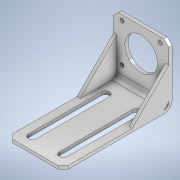
# Autodesk Inventor part: MotorBracket
Saved by Autodesk Inventor 2022 (Build 260153000, 153)
## iProperties
Created: 2022-09-25
Part Number: MotorBracket
Material: Stainless Steel
Document SubType Name: Modeling
Designer: adam
Density: 8 g/cm^3
Appearance: Aluminum - Dark
Mass: 392.424 g
Surface Area: 290.171 cm^2
Volume: 49.053 cm^3
Author: adam
Autodesk Inventor part; units mm, degrees
ref_plane "YZ Plane" through (0, 0, 0) normal (1, 0, 0) x (0, 1, 0)
ref_plane "XZ Plane" through (0, 0, 0) normal (0, 1, 0) x (-1, 0, 0)
ref_plane "XY Plane" through (0, 0, 0) normal (0, 0, 1) x (1, 0, 0)
sketch "Sketch1" plane through (0, 0, 0) normal (1, 0, 0) x (0, 1, 0)
  line L0 (0, 0) -> (4, 0)
  line L1 (4, 6) -> (4, 130)
  line L2 (4, 130) -> (0, 130)
  line L3 (0, 130) -> (0, 0)
  line L4 (10, 0) -> (74, 0)
  line L5 (74, 0) -> (74, -4)
  line L6 (74, -4) -> (10, -4)
  line L7 (0, 6) -> (0, 0)
  line L8 (4, 45) -> (49, 0)
  arc A0 (4, 6) -> (10, 0) centre (10, 6) ccw
  arc A1 (0, 6) -> (10, -4) centre (10, 6) ccw
  line L9 (4, 6) -> (10, 0)
  point P0 (0, -4)
  point P1 (0, 6)
  point P2 (2, 0)
  dimension "d0" = 4
  dimension "d1" = 130
  dimension "d2" = 70
  dimension "d3" = 45
  dimension "d4" = 45
  dimension "d35" = 10
  constraints: 20 end point, 6 point on line, 4 parallel, 4 point on circle, 4 tangent, 3 perpendicular, 2 centre point, 2 horizontal, 1 coincident
  measures "d0" distance of L4.end L5.end
  measures "d1" distance of L0.end L1.end
  measures "d2" distance from line of L4.end L1
  measures "d3" angle of L4 L8
  measures "d4" horizontal distance of L8.start L8.end
  measures "d35" radius of A1
extrude "Extrusion1" add sketch "Sketch1" along normal blind 68 contours A1 L3 L2 L1 A0 L4 L5 L6
extrude "Extrusion2" add sketch "Sketch1" along normal blind 4 contours L8 L4 L9 L1
extrude "Extrusion3" add sketch "Sketch1" against normal blind 4 from surface at 68 contours L8 L4 L9 L1
sketch "Sketch2" plane through (0, 74, 0) normal (0, 0, 1) x (1, 0, 0)
  line L0 (0, 0) -> (68, 0) construction
  line L1 (4, 0) -> (64, 0) construction
  line L2 (64, 0) -> (64, -60) construction
  line L3 (64, -60) -> (4, -60) construction
  line L4 (4, -60) -> (4, 0) construction
  line L5 (4, -25) -> (4, -70) construction
  line L6 (64, -70) -> (64, -25) construction
  line L7 (10.43, -6.43) -> (57.57, -6.43) construction
  line L8 (57.57, -6.43) -> (57.57, -53.57) construction
  line L9 (57.57, -53.57) -> (10.43, -53.57) construction
  line L10 (10.43, -53.57) -> (10.43, -6.43) construction
  line L11 (4, 0) -> (64, -60) construction
  line L12 (4, -60) -> (64, 0) construction
  circle A0 centre (34, -30) radius 20
  circle A1 centre (10.43, -6.43) radius 2.5
  circle A2 centre (57.57, -6.43) radius 2.5
  circle A3 centre (57.57, -53.57) radius 2.5
  circle A4 centre (10.43, -53.57) radius 2.5
  dimension "d26" = 60
  dimension "d27" = 60
  dimension "d28" = 47.14
  dimension "d29" = 40
  dimension "d30" = 5
  constraints: 20 end point, 5 centre point, 5 point on line, 4 parallel, 3 coincident, 3 equal radius, 2 collinear, 2 horizontal, 2 perpendicular, 1 midpoint
  measures "d26" distance between parallel lines of L0 L3
  measures "d27" distance between parallel lines of L2 L4
  measures "d28" distance of L7.start L7.end
  measures "d29" diameter of A0
  measures "d30" diameter of A1
extrude "Extrusion4" cut sketch "Sketch2" against normal through all
sketch "Sketch3" plane through (0, 4, 130) normal (0, 1, 0) x (1, 0, 0)
  line L0 (15, 15) -> (15, 105) construction
  line L1 (10, 15) -> (10, 105)
  line L2 (20, 105) -> (20, 15)
  arc A0 (10, 15) -> (20, 15) centre (15, 15) ccw
  arc A1 (20, 105) -> (10, 105) centre (15, 105) ccw
  line L3 (53, 15) -> (53, 105) construction
  line L4 (58, 15) -> (58, 105)
  line L5 (48, 105) -> (48, 15)
  arc A2 (48, 15) -> (58, 15) centre (53, 15) ccw
  arc A3 (58, 105) -> (48, 105) centre (53, 105) ccw
  line L6 (0, 0) -> (68, 0) projected
  line L7 (0, 85) -> (0, 0) projected
  line L8 (68, 85) -> (68, 0) projected
  point P0 (0, 130)
  point P1 (15, 60)
  point P2 (53, 60)
  dimension "d19" = 90
  dimension "d20" = 15
  dimension "d21" = 15
  dimension "d22" = 15
  dimension "d23" = 5
  constraints: 16 end point, 8 point on circle, 8 tangent, 4 centre point, 4 parallel, 2 midpoint, 1 equal radius, 1 horizontal alignment, 1 vertical
  measures "d19" distance of L1.start L1.end
  measures "d20" distance from line of L6 L0.start
  measures "d21" distance from line of L7 L0.start
  measures "d22" distance from line of L8 L3.start
  measures "d23" radius of A1
extrude "Extrusion5" cut sketch "Sketch3" against normal through all
chamfer "Chamfer1" distance 6 angle 45 4 edges at (68, 74, -2) (0, 74, -2) (68, 2, 130) (0, 2, 130)
ref_plane "Work Plane1" through (34, 0, 0) normal (1, 0, 0) x (0, 0, -1)
body "Solid1"
